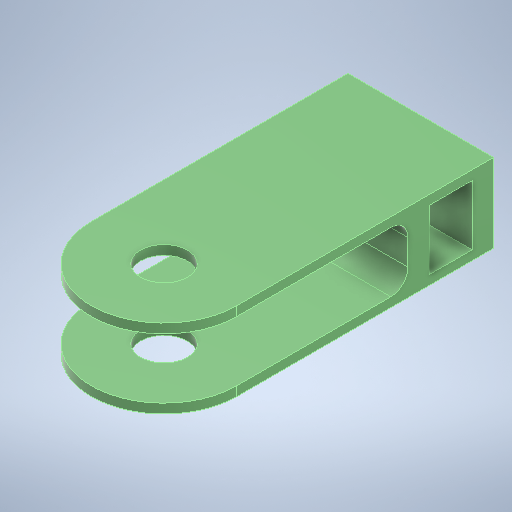
# Autodesk Inventor part: bielle sup
Saved by Autodesk Inventor 2026.2 (Build 302298010, 298A)
## iProperties
Created: 2026-03-17
Part Number: bielle sup
Material: Générique
Document SubType Name: Modeling
Designer: genon
Density: 1 g/cm^3
Appearance: Lisse - Vert forêt foncé
Author: genon
Autodesk Inventor part; units mm, degrees
ref_plane "YZ Plane" through (0, 0, 0) normal (1, 0, 0) x (0, 1, 0)
sketch "Esquisse1" plane through (0, 0, 0) normal (0, 1, 0) x (-1, 0, 0)
  circle A0 centre (0, 0) radius 8.5
  circle A1 centre (0, 0) radius 2.75
  line L0 (0, 0) -> (0, -30)
  line L1 (8.5, -30) -> (8.5, 0)
  line L2 (-8.5, -30) -> (-8.5, 0)
  line L3 (8.5, -30) -> (-8.5, -30)
  dimension "d0" = 17
  dimension "d1" = 5.5
  dimension "d4" = 30
  dimension "d5" = 30
  dimension "d6" = 30
  constraints: 8 end point, 2 centre point, 2 coincident, 2 point on circle, 2 tangent, 1 horizontal, 1 vertical
  measures "d0" diameter of A0
  measures "d1" diameter of A1
  measures "d4" distance of L0.start L0.end
  measures "d5" distance of L1.start L1.end
  measures "d6" distance of L2.start L2.end
extrude "Extrusion1" add sketch "Esquisse1" along normal blind 1.1
ref_plane "Plan de construction1" through (0, 8.1, 0) normal (0, 1, 0) x (1, 0, 0)
sketch "Esquisse3" plane through (0, 8.1, 0) normal (0, 1, 0) x (1, 0, 0)
  arc A0 (-8.5, 0) -> (8.5, 0) centre (0, 0) ccw projected
  line L0 (-8.5, 20) -> (-8.5, 0) projected
  line L1 (8.5, 0) -> (8.5, 20) projected
  line L2 (-8.5, 30) -> (-8.5, 15) projected
  line L3 (8.5, 30) -> (-8.5, 30) projected
  line L4 (8.5, 15) -> (8.5, 30) projected
  circle A1 centre (0, 0) radius 2.75 projected
extrude "Extrusion3" add sketch "Esquisse3" along normal blind 1.1
ref_plane "Plan de construction2" through (0, 4.6, 0) normal (0, -1, 0) x (1, 0, 0)
sketch "Esquisse7" plane through (0, 4.6, 0) normal (0, -1, 0) x (1, 0, 0)
  line L0 (8.5, -30) -> (-8.5, -30) projected
  line L1 (-8.5, -30) -> (8.5, -30)
  line L2 (8.5, -30) -> (8.5, -20)
  line L3 (8.5, -20) -> (-8.5, -20)
  line L4 (-8.5, -20) -> (-8.5, -30)
  point P0 (0, 0)
  dimension "d41" = 10
  constraints: 8 end point, 3 perpendicular, 1 collinear
  measures "d41" distance of L0.start L2.end
extrude "Extrusion5" add sketch "Esquisse7" along normal mid plane 7
sketch "Esquisse8" plane through (8.5, 0, 0) normal (1, 0, 0) x (0, 0, -1)
  line L0 (20, 8.1) -> (0, 8.1) projected
  line L1 (30, 0) -> (30, 9.2) projected
  line L2 (0, 0) -> (30, 0) projected
  line L3 (25, 8.1) -> (27.5, 8.1)
  line L4 (27.5, 8.1) -> (22.5, 8.1)
  line L5 (22.5, 8.1) -> (22.5, 1.1)
  line L6 (22.5, 1.1) -> (27.5, 1.1)
  line L7 (27.5, 1.1) -> (27.5, 8.1)
  line L8 (0, 9.2) -> (30, 9.2) projected
  dimension "d43" = 5
  dimension "d44" = 7
  dimension "d45" = 1.1
  dimension "d46" = 2.5
  constraints: 10 end point, 2 parallel, 1 horizontal, 1 perpendicular
  measures "d43" distance of L6.end L5.end
  measures "d44" distance of L5.end L4.end
  measures "d45" distance between parallel lines of L8 L3
  measures "d46" distance between parallel lines of L1 L7
extrude "Extrusion6" cut sketch "Esquisse8" against normal through all
sketch "Esquisse9" plane through (8.5, 0, -30) normal (0, 0, -1) x (-1, 0, 0)
  line L0 (5.75, 9.2) -> (11.25, 9.2) projected
  line L1 (8.5, 9.2) -> (8.5, 0)
  point P0 (8.5, 4.6)
  constraints: 2 end point, 2 midpoint, 1 vertical
hole "Perçage3" at (0, 4.6, -30) direction (0, 0, 1) diameter 5 end through all
fillet "Congé3" radius 2 2 edges at (0, 8.1, -20) (0, 1.1, -20)
